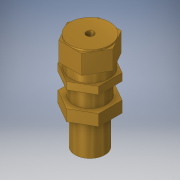
# Autodesk Inventor part: am-2002
Saved by Autodesk Inventor 2016 SP2 (Build 200236200, 236)
## iProperties
Created: 2017-03-28
Part Number: am-2002
Material: Brass
Document SubType Name: Modeling
Designer: smiku
Mass: 65.2751 g
Surface Area: 31.9771 cm^2
Volume: 7.68847 cm^3
Density: 8.49 g/cm^3
Appearance: Brass - Polished
Author: smiku
Autodesk Inventor part; units mm, degrees
ref_plane "YZ Plane" through (0, 0, 0) normal (1, 0, 0) x (0, 1, 0)
ref_plane "XZ Plane" through (0, 0, 0) normal (0, 1, 0) x (-1, 0, 0)
ref_plane "XY Plane" through (0, 0, 0) normal (0, 0, 1) x (1, 0, 0)
sketch "Sketch1" plane through (0, 0, 0) normal (0, 1, 0) x (-1, 0, 0)
  circle A0 centre (0, 0) radius 1.5875
  circle A1 centre (0, 0) radius 8.4963
  dimension "d0" = 3.175
  dimension "d1" = 16.9926
  constraints: 2 centre point, 2 coincident
  measures "d0" diameter of A0
  measures "d1" diameter of A1
extrude "Extrusion1" add sketch "Sketch1" against normal blind 0.7112
sketch "Sketch2" plane through (0, -0.7112, 0) normal (0, -1, 0) x (1, 0, 0)
  circle A0 centre (0, 0) radius 8.4963 construction
  line L0 (4.9053, 8.4963) -> (9.8107, 0)
  line L1 (9.8107, 0) -> (4.9053, -8.4963)
  line L2 (4.9053, -8.4963) -> (-4.9053, -8.4963)
  line L3 (-4.9053, -8.4963) -> (-9.8107, 0)
  line L4 (-9.8107, 0) -> (-4.9053, 8.4963)
  line L5 (-4.9053, 8.4963) -> (4.9053, 8.4963)
  circle A1 centre (0, 0) radius 1.5875 projected
  point P0 (0, 8.4963)
  constraints: 12 end point, 1 coincident, 1 horizontal, 1 midpoint, 1 vertical alignment, 14 other
extrude "Extrusion2" add sketch "Sketch2" along normal blind 8.1534
sketch "Sketch3" plane through (0, -8.8646, 0) normal (0, -1, 0) x (1, 0, 0)
  circle A0 centre (0, 0) radius 8.2296
  dimension "d6" = 16.4592
  constraints: 1 centre point, 1 coincident
  measures "d6" diameter of A0
extrude "Extrusion3" add sketch "Sketch3" along normal blind 3.81
sketch "Sketch4" plane through (0, -12.6746, 0) normal (0, -1, 0) x (1, 0, 0)
  circle A0 centre (0, 0) radius 8.7249 construction
  line L0 (8.7249, -5.0373) -> (0, -10.0746)
  line L1 (0, -10.0746) -> (-8.7249, -5.0373)
  line L2 (-8.7249, -5.0373) -> (-8.7249, 5.0373)
  line L3 (-8.7249, 5.0373) -> (0, 10.0746)
  line L4 (0, 10.0746) -> (8.7249, 5.0373)
  line L5 (8.7249, 5.0373) -> (8.7249, -5.0373)
  point P0 (8.7249, 0)
  dimension "d9" = 17.4498
  constraints: 12 end point, 2 coincident, 1 horizontal alignment, 1 midpoint, 1 vertical, 15 other
extrude "Extrusion4" add sketch "Sketch4" along normal blind 3.175
sketch "Sketch5" plane through (0, -15.8496, 0) normal (0, -1, 0) x (1, 0, 0)
  circle A0 centre (0, 0) radius 7.112
  dimension "d12" = 14.224
  constraints: 1 centre point, 1 coincident
  measures "d12" diameter of A0
extrude "Extrusion5" add sketch "Sketch5" along normal blind 6.985
sketch "Sketch6" plane through (0, -22.8346, 0) normal (0, -1, 0) x (1, 0, 0)
  circle A0 centre (0, 0) radius 8.7122 construction
  line L0 (8.7122, -5.03) -> (0, -10.06)
  line L1 (0, -10.06) -> (-8.7122, -5.03)
  line L2 (-8.7122, -5.03) -> (-8.7122, 5.03)
  line L3 (-8.7122, 5.03) -> (0, 10.06)
  line L4 (0, 10.06) -> (8.7122, 5.03)
  line L5 (8.7122, 5.03) -> (8.7122, -5.03)
  point P0 (8.7122, 0)
  dimension "d15" = 17.4244
  constraints: 12 end point, 2 coincident, 1 horizontal alignment, 1 midpoint, 1 vertical, 15 other
extrude "Extrusion6" add sketch "Sketch6" along normal blind 4.8514
sketch "Sketch7" plane through (0, -27.686, 0) normal (0, -1, 0) x (1, 0, 0)
  circle A0 centre (0, 0) radius 2.4765
  circle A1 centre (0, 0) radius 6.35
  dimension "d18" = 4.953
  dimension "d19" = 12.7
  constraints: 2 centre point, 2 coincident
  measures "d18" diameter of A0
  measures "d19" diameter of A1
extrude "Extrusion7" add sketch "Sketch7" along normal blind 14.1986
body "Solid1"
